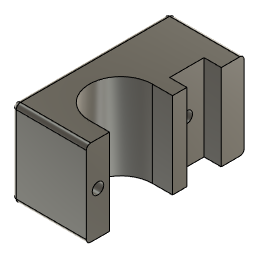
ConectorEstruturaGK_ampliado (Autodesk Fusion 360 design; units mm, degrees)
Autodesk Fusion 360 part; units mm, degrees
sketch "Esboço1" plane through (0, 0, 0) normal (0, 0, 1) x (1, 0, 0)
  arc A0 (21, 37) -> (21, 15) centre (21, 26) ccw
  line L0 (1.9999, 62) -> (2, 62)
  line L1 (2, 7) -> (2, 62)
  line L2 (21, 37) -> (28, 37)
  line L3 (28, 37) -> (28, 42)
  line L4 (28, 42) -> (22, 42)
  line L5 (22, 42) -> (22, 54)
  line L6 (22, 54) -> (28, 54)
  line L7 (28, 54) -> (28, 62)
  line L8 (28, 62) -> (1.9999, 62)
  line L9 (21, 15) -> (28, 15)
  line L10 (28, 15) -> (28, 6.9481)
  line L11 (28, 6.9481) -> (2, 7)
  dimension "d13" = 11
  dimension "d18" = 6
  dimension "d19" = 12
  dimension "d21" = 8
  constraint tangent A0 L2
  constraint horizontal L2
  constraint vertical L3
  constraint coincident L2.end L3.start
  constraint perpendicular L3 L4
  constraint perpendicular L4 L5
  constraint perpendicular L5 L6
  constraint perpendicular L6 L7
  constraint tangent A0 L9
  constraint perpendicular L9 L10
  measures "d13" distance of A0.start A0.centre
  measures "d18" distance of L3.end L4.end
  measures "d19" distance of L4.end L5.end
  measures "d21" distance of L6.end L7.end
extrude "Extrusão1" add sketch "Esboço1" along normal blind 30
hole "Furo1" at (2, 48, 15) direction (1, 0, 0) diameter 4 depth 40 tip angle 180
hole "Furo2" at (2, 11, 15) direction (1, 0, 0) diameter 4 depth 40 tip angle 180
fillet "Arredondamento1" radius 1.5 8 edges at (2, 34.5, 30) (15, 6.9741, 30) (2, 7, 15) (15, 6.9741, 0) (2, 34.5, 0) (2, 62, 15) (15, 62, 0) (15, 62, 30)
sketch "Esboço2" plane through (2, 0, 0) normal (-1, 0, 0) x (0, -1, 0)
  circle A0 centre (-48, 15) radius 2
  circle A1 centre (-11, 15) radius 2
  line L0 (-60.5, 1.5) -> (-8.497, 1.5)
  line L1 (-8.497, 1.5) -> (-8.497, 28.5)
  line L2 (-8.497, 28.5) -> (-60.5, 28.5)
  line L3 (-60.5, 28.5) -> (-60.5, 1.5)
  circle A2 centre (-48, 15) radius 5
  constraint concentric A0 A2
extrude "Extrusão2" cut sketch "Esboço2" against normal blind 15 contours A2
